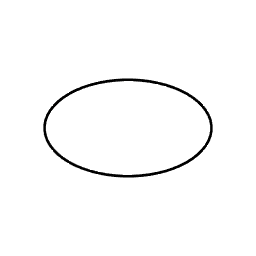
Rubber_118mm (Autodesk Fusion 360 design; units mm, degrees)
Autodesk Fusion 360 part; units mm, degrees
sketch "Sketch1" plane through (0, 0, 0) normal (0, 0, 1) x (1, 0, 0)
  circle A0 centre (0, 0) radius 59.2
  circle A1 centre (0, 0) radius 57.8
  dimension "d1" = 118.4
  dimension "d2" = 115.6
  constraint coincident A0.centre A1.centre
  measures "d1" diameter of A0
  measures "d2" diameter of A1
extrude "Extrude1" add sketch "Sketch1" along normal blind 0.6
fillet "Fillet1" radius 0.3 4 edges at (-55.1938, -21.4076, 0.6) (-55.1938, -21.4076, 0) (-53.8885, 20.9014, 0.6) (-53.8885, 20.9014, 0)
equation "d1 = outerDiameter"
equation "d2 = innerDiameter"
equation "d3 = height"
equation "d6 = height / 2"
equation "outerDiameter = 118.4 mm"
equation "innerDiameter = 115.6 mm"
equation "height = 0.6 mm"
named bodies: "Rubber_118mm"
